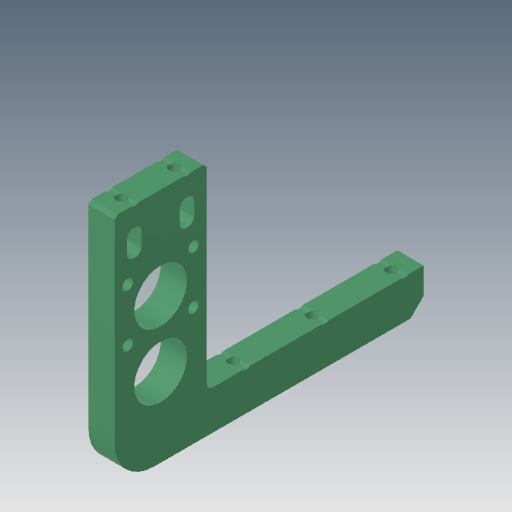
# Autodesk Inventor part: handle
Saved by Autodesk Inventor 2018 (Build 220112000, 112)
## iProperties
Created: 2018-09-01
Part Number: handle
Material: 一般
Document SubType Name: Modeling
Designer: y6tada
Density: 1 g/cm^3
Appearance: 滑らか - 濃い海緑
Author: y6tada
Autodesk Inventor part; units mm, degrees
ref_plane "YZ Plane" through (0, 0, 0) normal (1, 0, 0) x (0, 1, 0)
ref_plane "XZ Plane" through (0, 0, 0) normal (0, 1, 0) x (-1, 0, 0)
ref_plane "XY Plane" through (0, 0, 0) normal (0, 0, 1) x (1, 0, 0)
sketch "スケッチ1" plane through (0, 0, 0) normal (1, 0, 0) x (0, 1, 0)
  line L0 (0, 12) -> (0, -12) construction
  arc A0 (0, 0.6) -> (0, -0.6) centre (0.8, 0) ccw
  arc A1 (0, -11.4) -> (0, -12.6) centre (0.8, -12) ccw
  arc A2 (0, 12.6) -> (0, 11.4) centre (0.8, 12) ccw
  line L1 (0, 11.4) -> (0, 0.6)
  line L2 (0, -0.6) -> (0, -11.4)
  line L3 (0, -12.6) -> (0, -15)
  line L4 (0, -15) -> (-4, -15)
  line L5 (-4, -15) -> (-6, -13)
  line L6 (-6, -13) -> (-6, 26)
  line L7 (0, 32) -> (29.5, 32)
  line L8 (0, 12.6) -> (0, 17)
  line L9 (1, 18) -> (29.5, 18)
  arc A3 (1, 18) -> (0, 17) centre (1, 17) ccw
  line L10 (0.8, 12) -> (0.8, -12) construction
  arc A4 (0, 32) -> (-6, 26) centre (0, 26) ccw
  line L11 (30, 18.5) -> (30, 20.4)
  line L12 (30, 31.5) -> (29.5, 32)
  line L13 (30, 18.5) -> (29.5, 18)
  arc A5 (30, 29.6) -> (30, 28.4) centre (30.8, 29) ccw
  arc A6 (30, 21.6) -> (30, 20.4) centre (30.8, 21) ccw
  line L14 (30.8, 29) -> (30.8, 21) construction
  line L15 (30, 29.6) -> (30, 31.5)
  line L16 (30, 28.4) -> (30, 29.6) construction
  line L17 (30, 21.6) -> (30, 28.4)
  line L18 (30, 20.4) -> (30, 21.6) construction
  line L19 (30.8, 25) -> (24.681, 25) construction
  line L20 (26, 30.1) -> (24, 30.1)
  line L21 (23, 29.1) -> (23, 28.9)
  line L22 (24, 27.9) -> (26, 27.9)
  line L23 (27, 28.9) -> (27, 29.1)
  arc A7 (27, 29.1) -> (26, 30.1) centre (26, 29.1) ccw
  arc A8 (26, 27.9) -> (27, 28.9) centre (26, 28.9) ccw
  arc A9 (23, 28.9) -> (24, 27.9) centre (24, 28.9) ccw
  arc A10 (24, 30.1) -> (23, 29.1) centre (24, 29.1) ccw
  line L24 (27, 29) -> (30.8, 29) construction
  line L25 (26, 19.9) -> (24, 19.9)
  line L26 (23, 20.9) -> (23, 21.1)
  line L27 (24, 22.1) -> (26, 22.1)
  line L28 (27, 21.1) -> (27, 20.9)
  arc A11 (26, 19.9) -> (27, 20.9) centre (26, 20.9) ccw
  arc A12 (27, 21.1) -> (26, 22.1) centre (26, 21.1) ccw
  arc A13 (24, 22.1) -> (23, 21.1) centre (24, 21.1) ccw
  arc A14 (23, 20.9) -> (24, 19.9) centre (24, 20.9) ccw
  line L29 (20, 30) -> (12, 30) construction
  line L30 (12, 30) -> (12, 20) construction
  line L31 (12, 20) -> (20, 20) construction
  line L32 (20, 20) -> (20, 30) construction
  circle A15 centre (20, 30) radius 0.8
  circle A16 centre (20, 20) radius 0.8
  circle A17 centre (12, 20) radius 0.8
  circle A18 centre (12, 30) radius 0.8
  line L33 (20, 30) -> (12, 20) construction
  circle A19 centre (16, 25) radius 4
  line L34 (16, 25) -> (6, 25) construction
  circle A20 centre (6, 25) radius 4
  point P0 (0, 0)
  point P1 (0, 0)
  point P2 (30, 32)
  point P3 (30, 18)
  point P4 (27, 21)
  dimension "d0" = 24
  dimension "d1" = 1
  dimension "d2" = 0.8
  dimension "d3" = 1
  dimension "d4" = 6
  dimension "d5" = 2
  dimension "d6" = 3
  dimension "d7" = 2
  dimension "d8" = 6
  dimension "d11" = 6
  dimension "d31" = 0.5
  dimension "d32" = 0.5
  dimension "d33" = 0.5
  dimension "d34" = 0.5
  dimension "d35" = 30
  dimension "d36" = 14
  dimension "d37" = 1
  dimension "d38" = 0.8
  dimension "d39" = 8
  dimension "d40" = 1
  dimension "d41" = 3
  dimension "d42" = 4
  dimension "d43" = 2.2
  dimension "d44" = 1.6
  dimension "d45" = 10
  dimension "d46" = 8
  dimension "d47" = 10
  dimension "d48" = 10
  constraints: 70 end point, 30 point on circle, 21 centre point, 13 symmetric about line, 13 tangent, 10 equal radius, 9 point on line, 9 vertical, 6 coincident, 6 parallel, 5 horizontal, 5 midpoint, 4 perpendicular, 3 horizontal alignment, 2 collinear, 6 other
  measures "d0" distance of L0.start L0.end
  measures "d1" radius of A3
  measures "d2" distance between parallel lines of L0 L10
  measures "d3" radius of A2
  measures "d4" distance between parallel lines of L6 L3
  measures "d5" distance from line of L6 L4.end
  measures "d6" distance from line of L10.end L4
  measures "d7" distance from line of L4 L5.end
  measures "d8" distance from line of L10.start L9
  measures "d11" radius of A4
  measures "d31" distance of L12.start point (30, 32)
  measures "d32" distance of L7.end point (30, 32)
  measures "d33" distance of L11.start point (30, 18)
  measures "d34" distance of L9.end point (30, 18)
  measures "d35" distance from line of point (0, 0) L11
  measures "d36" distance between parallel lines of L7 L9
  measures "d37" radius of A5
  measures "d38" distance between parallel lines of L11 L14
  measures "d39" distance of L14.start L14.end
  measures "d40" radius of A7
  measures "d41" distance between parallel lines of L23 L16
  measures "d42" distance between parallel lines of L21 L23
  measures "d43" distance between parallel lines of L20 L22
  measures "d44" diameter of A16
  measures "d45" distance between parallel lines of L17 L32
  measures "d46" distance of L30.end L31.end
  measures "d47" distance between parallel lines of L29 L31
  measures "d48" distance of L34.start L34.end
extrude "押し出し1" add sketch "スケッチ1" along normal mid plane 4
sketch "スケッチ2" plane through (-2, 0, 11.4) normal (0, 1, 0) x (1, 0, 0)
  circle A0 centre (2, 11.4) radius 0.8
  line L0 (4, -1.2) -> (0, -1.2) construction
  line L1 (4, 0) -> (0, 0) construction
  line L2 (0, -1.2) -> (4, 0) construction
  circle A1 centre (2, -0.6) radius 0.8
  line L3 (4, 22.8) -> (0, 22.8) construction
  line L4 (4, 24) -> (0, 24) construction
  line L5 (0, 22.8) -> (4, 24) construction
  circle A2 centre (2, 23.4) radius 0.8
  dimension "d14" = 1.6
  constraints: 4 end point, 3 centre point, 2 equal radius, 2 midpoint, 1 coincident
  measures "d14" diameter of A1
extrude "押し出し2" cut sketch "スケッチ2" against normal blind 6
sketch "スケッチ4" plane through (-2, 30, 28.4) normal (0, 1, 0) x (1, 0, 0)
  line L0 (4, -1.2) -> (0, -1.2) construction
  line L1 (4, 0) -> (0, 0) construction
  line L2 (0, -1.2) -> (4, 0) construction
  line L3 (4, 6.8) -> (0, 6.8) construction
  line L4 (4, 8) -> (0, 8) construction
  line L5 (0, 6.8) -> (4, 8) construction
  circle A0 centre (2, -0.6) radius 0.8
  circle A1 centre (2, 7.4) radius 0.8
  point P0 (2, 28.4)
  dimension "d49" = 1.6
  constraints: 4 end point, 2 centre point, 2 midpoint, 1 equal radius
  measures "d49" diameter of A0
extrude "押し出し4" cut sketch "スケッチ4" against normal blind 5
equation "\"d32\" = d31"
equation "\"d33\" = d31"
equation "\"d34\" = d33"
